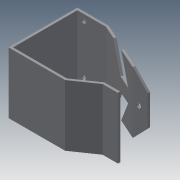
# Autodesk Inventor part: kryt_ruka
Saved by Autodesk Inventor 2013 (Build 170138000, 138)
## iProperties
Created: 2013-02-06
Part Number: kryt_ruka
Material: Generic
Document SubType Name: Modeling
Designer: idle-rug
Density: 1 g/cm^3
Author: idle-rug
Autodesk Inventor part; units mm, degrees
ref_plane "YZ Plane" through (0, 0, 0) normal (1, 0, 0) x (0, 1, 0)
ref_plane "XZ Plane" through (0, 0, 0) normal (0, 1, 0) x (-1, 0, 0)
ref_plane "XY Plane" through (0, 0, 0) normal (0, 0, 1) x (1, 0, 0)
sketch "Sketch1" plane through (0, 0, 0) normal (0, 1, 0) x (-1, 0, 0)
  line L0 (-9.5, 20) -> (9.5, 20)
  line L1 (9.5, 20) -> (9.5, -20)
  line L2 (9.5, -20) -> (-9.5, -20)
  line L3 (-9.5, -20) -> (-9.5, 20)
  line L4 (-9.5, 20) -> (9.5, -20) construction
  line L5 (9.5, 20) -> (-9.5, -20) construction
  point P0 (0, 0)
  dimension "d0" = 19
  dimension "d1" = 40
  constraints: 12 end point, 2 midpoint, 2 parallel, 1 horizontal, 1 perpendicular
  measures "d0" distance of L1.end L2.end
  measures "d1" distance of L0.end L1.end
extrude "Extrusion1" add sketch "Sketch1" along normal blind 1.5
sketch "Sketch2" plane through (-9.5, 0, 20) normal (0, 0, 1) x (1, 0, 0)
  line L0 (19, 0) -> (0, 0) projected
  line L1 (0, 0) -> (0, 1.5) projected
  line L2 (0, 0) -> (0, -22)
  line L3 (0, -22) -> (60, -22)
  line L4 (60, -22) -> (60, -14)
  line L5 (60, -14) -> (50, -14)
  line L6 (60, -12.357) -> (60, -14)
  line L7 (50, -12.357) -> (50, -14)
  line L8 (19, 1.5) -> (50, -12.357)
  line L9 (18.68, 0) -> (50, -14)
  line L10 (19, 1.5) -> (19, 0)
  line L11 (19, 0) -> (18.68, 0)
  line L12 (60, -14) -> (60, -12.5)
  line L13 (60, -12.5) -> (50, -12.5)
  line L14 (50, -12.357) -> (50.32, -12.5)
  line L15 (50.32, -12.5) -> (50.32, -14)
  line L16 (50, -14) -> (50.32, -14)
  point P0 (9.5, 0)
  dimension "d4" = 22
  dimension "d5" = 60
  dimension "d6" = 8
  dimension "d7" = 10
  dimension "d12" = 1.5
  constraints: 30 end point, 5 perpendicular, 5 point on line, 4 collinear, 2 parallel
  measures "d4" distance of L0.end L2.end
  measures "d5" distance of L2.end L3.end
  measures "d6" distance of L3.end L4.end
  measures "d7" distance of L4.end L5.end
  measures "d12" distance of L4.end L12.end
extrude "Extrusion2" add sketch "Sketch2" against normal blind 40 contours L10 L8 L7 L9 L0 | L7 L13 L15 L5 | L14 L13 L7 | L15 L13 L6 L5
sketch "Sketch3" plane through (40.82, -12.5, 20) normal (0.4080849, 0.912944, 0) x (0.912944, -0.4080849, 0)
  line L0 (0, 0) -> (-34.3066, 0) projected
  line L1 (-34.3066, 40) -> (0, 40) projected
  line L2 (-24.3066, 0) -> (-15.3066, 15.5885)
  line L3 (-24.3066, 0) -> (-6.3066, 0) construction
  line L4 (-15.3066, 15.5885) -> (-5.3066, 15.5885)
  line L5 (-5.3066, 15.5885) -> (-14.3066, 0)
  line L6 (-24.3066, 40) -> (-15.3066, 24.4115)
  line L7 (-24.3066, 40) -> (-6.3066, 40) construction
  line L8 (-15.3066, 24.4115) -> (-5.3066, 24.4115)
  line L9 (-5.3066, 24.4115) -> (-14.3066, 40)
  point P0 (-42.3674, 20)
  dimension "d15" = 10
  dimension "d16" = 18
  dimension "d17" = 60
  dimension "d18" = 10
  dimension "d21" = 18
  dimension "d22" = 60
  dimension "d23" = 10
  constraints: 16 end point, 4 point on line, 3 parallel, 2 equal length, 2 horizontal
  measures "d15" distance of L1.start L6.start
  measures "d16" distance of L2.start L2.end
  measures "d17" angle of L3 L2
  measures "d18" distance of L2.end L4.end
  measures "d21" distance of L6.start L6.end
  measures "d22" angle of L6 L7
  measures "d23" distance of L6.end L8.end
extrude "Extrusion3" cut sketch "Sketch3" against normal blind 1.5
sketch "Sketch4" plane through (40.82, -12.5, 20) normal (0, 1, 0) x (1, 0, 0)
  line L0 (9.68, 0) -> (0, 0) projected
  line L1 (9.68, 0) -> (9.68, 40) projected
  line L2 (0, 40) -> (9.68, 40) projected
  line L3 (9.68, 20) -> (4.84, 20)
  circle A0 centre (4.84, 20) radius 1.5
  line L4 (9.68, 20) -> (9.68, 10)
  line L5 (9.68, 10) -> (0, 0)
  line L6 (9.68, 20) -> (9.68, 30)
  line L7 (9.68, 30) -> (0, 40)
  line L8 (9.68, 10) -> (9.68, 0)
  line L9 (0, 0) -> (9.68, 0)
  line L10 (0, 0) -> (9.68, 10)
  line L11 (9.68, 40) -> (9.68, 30)
  line L12 (0, 40) -> (9.68, 40)
  line L13 (0, 40) -> (9.68, 30)
  point P0 (-40.82, 20)
  dimension "d26" = 3
  dimension "d27" = 10
  dimension "d28" = 10
  constraints: 22 end point, 4 collinear, 2 point on line, 1 centre point, 1 coincident, 1 midpoint, 1 perpendicular
  measures "d26" diameter of A0
  measures "d27" distance of L3.start L4.end
  measures "d28" distance of L3.start L6.end
extrude "Extrusion4" cut sketch "Sketch4" against normal blind 1.5 contours L0 L5 L1 | L7 L2 L1
sketch "Sketch8" plane through (40.82, -12.5, 20) normal (0, 1, 0) x (1, 0, 0)
  circle A0 centre (4.84, 20) radius 1.5
  point P0 (-40.82, 20)
  dimension "d31" = 3
  constraints: 1 centre point
  measures "d31" diameter of A0
extrude "Extrusion5" cut sketch "Sketch8" against normal blind 1.5
sketch "Sketch9" plane through (0, 1.5, 0) normal (0, 1, 0) x (1, 0, 0)
  line L0 (-9.5, 20) -> (-5.5, 20)
  line L1 (-9.5, 16) -> (-9.5, 20)
  line L2 (-9.5, -20) -> (-5.5, -20)
  line L3 (-9.5, -16) -> (-9.5, -20)
  circle A0 centre (-5.5, -16) radius 1.5
  circle A1 centre (-5.5, 16) radius 1.5
  point P0 (0, 0)
  dimension "d38" = 3
  dimension "d39" = 3
  constraints: 8 end point, 2 centre point, 2 horizontal
  measures "d38" diameter of A0
  measures "d39" diameter of A1
extrude "Extrusion6" cut sketch "Sketch9" against normal blind 1.5
sketch "Sketch10" plane through (40.82, -12.5, 20) normal (0, 1, 0) x (1, 0, 0)
  circle A0 centre (4.84, 20) radius 1.5 projected
extrude "Extrusion7" add sketch "Sketch10" against normal blind 1.5
sketch "Sketch11" plane through (40.82, -12.5, 20) normal (0, 1, 0) x (1, 0, 0)
  line L0 (9.68, 10) -> (9.68, 30) projected
  line L1 (0, 0) -> (0, 40) projected
  line L2 (9.68, 20) -> (3.68, 20)
  circle A0 centre (3.68, 20) radius 1.5
  dimension "d44" = 6
  dimension "d45" = 3
  constraints: 2 end point, 1 centre point, 1 coincident, 1 midpoint, 1 perpendicular
  measures "d44" distance of L2.start L2.end
  measures "d45" diameter of A0
extrude "Extrusion8" cut sketch "Sketch11" against normal blind 1.5
sketch "Sketch12" plane through (0, 1.5, 0) normal (0, 1, 0) x (1, 0, 0)
  line L0 (-9.5, 20) -> (-9.5, -20) projected
  line L1 (-9.5, 20) -> (-9.5, -20)
  line L2 (-9.5, -20) -> (-11, -20)
  line L3 (-11, -20) -> (-11, 20)
  line L4 (-11, 20) -> (-9.5, 20)
  point P0 (0, 0)
  dimension "d48" = 1.5
  constraints: 8 end point, 2 equal length, 2 perpendicular
  measures "d48" distance of L0.end L2.end
extrude "Extrusion9" add sketch "Sketch12" against normal blind 38
sketch "Sketch13" plane through (-11, 1.5, -20) normal (-1, 0, 0) x (0, 0, 1)
  line L0 (40, -38) -> (0, -38) projected
  line L1 (0, -38) -> (40, -38)
  line L2 (40, -38) -> (40, -39.5)
  line L3 (40, -39.5) -> (0, -39.5)
  line L4 (0, -38) -> (0, -39.5)
  point P0 (20, -1.5)
  dimension "d51" = 1.5
  constraints: 8 end point, 3 perpendicular, 1 collinear
  measures "d51" distance of L0.start L2.end
extrude "Extrusion10" add sketch "Sketch13" against normal blind 1.5
sketch "Sketch15" plane through (-11, -38, -20) normal (0, -1, 0) x (1, 0, 0)
  line L0 (0, 0) -> (0, 40) projected
  line L1 (0, 0) -> (1.5, 0) projected
  line L2 (1.5, 40) -> (1.5, 0) projected
  line L3 (0, 40) -> (1.5, 40) projected
  point P0 (11, 20)
extrude "Extrusion11" add sketch "Sketch15" along normal blind 4
sketch "Sketch16" plane through (-11, 1.5, -20) normal (-1, 0, 0) x (0, 0, 1)
  line L0 (0, 0) -> (0, -43.5) projected
  line L1 (40, -43.5) -> (0, -43.5) projected
  line L2 (40, 0) -> (40, -43.5) projected
  line L3 (0, -43.5) -> (0, -42)
  line L4 (0, -42) -> (40, -42)
  line L5 (40, -42) -> (40, -43.5)
  line L6 (40, -43.5) -> (0, -43.5)
  line L7 (40, -43.5) -> (40, -45)
  line L8 (40, -45) -> (0, -45)
  line L9 (0, -43.5) -> (0, -45)
  point P0 (20, -1.5)
  dimension "d56" = 1.5
  dimension "d57" = 1.5
  constraints: 14 end point, 5 perpendicular, 2 point on line, 1 collinear
  measures "d56" distance of L0.end L3.end
  measures "d57" distance of L1.start L7.end
extrude "Extrusion12" add sketch "Sketch16" against normal blind 37 contours L1 L7 L8 L9
sketch "Sketch17" plane through (9.18, 0, -20) normal (0, 0, -1) x (-1, 0, 0)
  line L0 (18.68, 0) -> (18.68, -42) projected
  line L1 (18.68, -42) -> (-16.82, -42) projected
  line L2 (-16.82, -43.5) -> (-16.82, -42) projected
  line L3 (18.68, -42) -> (18.68, -24)
  line L4 (18.68, -24) -> (-41.32, -24)
  line L5 (-41.32, -24) -> (-41.32, -32)
  line L6 (-41.32, -32) -> (-31.32, -32)
  line L7 (-31.32, -32) -> (-31.32, -33.5)
  line L8 (-31.32, -33.5) -> (-41.32, -33.5)
  line L9 (-41.32, -33.5) -> (-41.32, -32)
  line L10 (-16.82, -43.5) -> (-31.32, -33.5)
  line L11 (-31.32, -32) -> (-30.8529, -32)
  line L12 (-30.8529, -32) -> (-16.3529, -42)
  line L13 (-16.3529, -42) -> (-16.82, -42)
  line L14 (-16.82, -42) -> (-16.82, -43.5)
  point P0 (9.18, 0)
  dimension "d60" = 18
  dimension "d61" = 60
  dimension "d62" = 8
  dimension "d63" = 10
  dimension "d64" = 1.5
  constraints: 24 end point, 5 perpendicular, 3 collinear, 3 point on line, 1 parallel
  measures "d60" distance of L0.end L3.end
  measures "d61" distance of L3.end L4.end
  measures "d62" distance of L4.end L5.end
  measures "d63" distance of L5.end L6.end
  measures "d64" distance of L6.end L7.end
extrude "Extrusion13" add sketch "Sketch17" against normal blind 40 contours L1 L2 L10 L7 L11 L12 | L6 L7 L8 L9
body "Solid1"
